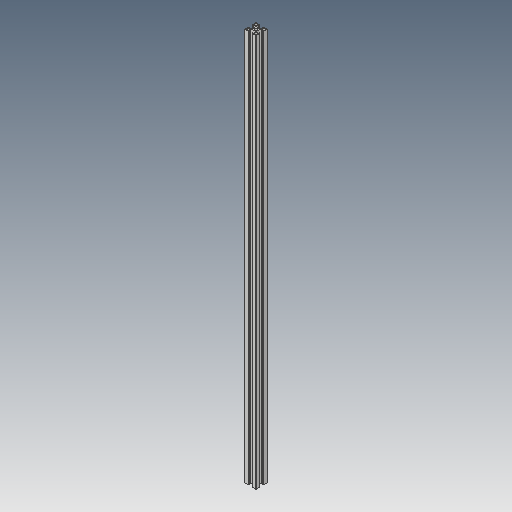
# Autodesk Inventor part: Propile_202070
Saved by Autodesk Inventor 2019 (Build 230136000, 136)
## iProperties
Created: 2019-05-03
Part Number: Propile_202070
Material: 일반
Document SubType Name: Modeling
Designer: hinmo
Density: 1 g/cm^3
Appearance: 기본값
Author: hinmo
Autodesk Inventor part; units mm, degrees
ref_plane "YZ Plane" through (0, 0, 0) normal (1, 0, 0) x (0, 1, 0)
ref_plane "XZ Plane" through (0, 0, 0) normal (0, 1, 0) x (-1, 0, 0)
ref_plane "XY Plane" through (0, 0, 0) normal (0, 0, 1) x (1, 0, 0)
sketch "스케치1" plane through (0, 0, 0) normal (0, 1, 0) x (-1, 0, 0)
  line L0 (10, 10) -> (-10, 10)
  line L1 (-10, 10) -> (-10, -10)
  line L2 (-10, -10) -> (10, -10)
  line L3 (10, -10) -> (10, 10)
  line L4 (10, 10) -> (-10, -10) construction
  line L5 (-10, 10) -> (10, -10) construction
  circle A0 centre (0, 0) radius 2.15
  line L6 (-10, 0) -> (-10, 2.65)
  line L7 (-10, 2.65) -> (-8.5, 2.65)
  line L8 (-8.5, 2.65) -> (-8.5, 4.15)
  line L9 (-8.5, 4.15) -> (-5, 4.15)
  line L10 (7, 7) -> (-7, -7) construction
  line L11 (-7, 7) -> (7, -7) construction
  circle A1 centre (-7, -7) radius 2
  circle A2 centre (-7, 7) radius 2
  circle A3 centre (7, 7) radius 2
  circle A4 centre (7, -7) radius 2
  line L12 (0, -10) -> (0, 0)
  line L13 (-10, 0) -> (-10, -2.65)
  line L14 (-10, -2.65) -> (-8.5, -2.65)
  line L15 (-8.5, -2.65) -> (-8.5, -4.15)
  line L16 (-8.5, -4.15) -> (-5, -4.15)
  arc A5 (-5, -4.15) -> (-5, 4.15) centre (-10.26, 0) ccw
  line L17 (0, 10) -> (2.65, 10)
  line L18 (2.65, 10) -> (2.65, 8.5)
  line L19 (2.65, 8.5) -> (4.15, 8.5)
  line L20 (4.15, 8.5) -> (4.15, 5)
  line L21 (0, 10) -> (-2.65, 10)
  line L22 (-2.65, 10) -> (-2.65, 8.5)
  line L23 (-2.65, 8.5) -> (-4.15, 8.5)
  line L24 (-4.15, 8.5) -> (-4.15, 5)
  arc A6 (-4.15, 5) -> (4.15, 5) centre (0, 10.26) ccw
  line L25 (8.5, -2.65) -> (8.5, -4.15)
  line L26 (10, 0) -> (10, -2.65)
  line L27 (8.5, -4.15) -> (5, -4.15)
  arc A7 (5, 4.15) -> (5, -4.15) centre (10.26, 0) ccw
  line L28 (10, -2.65) -> (8.5, -2.65)
  line L29 (8.5, 4.15) -> (5, 4.15)
  line L30 (8.5, 2.65) -> (8.5, 4.15)
  line L31 (10, 0) -> (10, 2.65)
  line L32 (10, 2.65) -> (8.5, 2.65)
  line L33 (-4.15, -8.5) -> (-4.15, -5)
  line L34 (4.15, -8.5) -> (4.15, -5)
  line L35 (2.65, -8.5) -> (4.15, -8.5)
  line L36 (-2.65, -8.5) -> (-4.15, -8.5)
  line L37 (0, -10) -> (2.65, -10)
  line L38 (2.65, -10) -> (2.65, -8.5)
  line L39 (0, -10) -> (-2.65, -10)
  line L40 (-2.65, -10) -> (-2.65, -8.5)
  arc A8 (4.15, -5) -> (-4.15, -5) centre (0, -10.26) ccw
  dimension "d6" = 20
  dimension "d7" = 20
  dimension "d8" = 4.3
  dimension "d9" = 2.65
  dimension "d10" = 1.5
  dimension "d11" = 1.5
  dimension "d12" = 3.5
  dimension "d13" = 14
  dimension "d14" = 14
  dimension "d15" = 4
  dimension "d16" = 4
  dimension "d17" = 4
  dimension "d18" = 4
  dimension "d22" = 2.65
  dimension "d23" = 1.5
  dimension "d24" = 3.5
  dimension "d25" = 6.7
  dimension "d26" = 1.5
  dimension "d27" = 2.65
  dimension "d28" = 1.5
  dimension "d29" = 1.5
  dimension "d30" = 3.5
  dimension "d31" = 2.65
  dimension "d32" = 1.5
  dimension "d33" = 3.5
  dimension "d34" = 6.7
  dimension "d35" = 1.5
  dimension "d36" = 2.65
  dimension "d37" = 1.5
  dimension "d38" = 1.5
  dimension "d39" = 3.5
  dimension "d40" = 2.65
  dimension "d41" = 1.5
  dimension "d42" = 3.5
  dimension "d43" = 6.7
  dimension "d44" = 1.5
  dimension "d45" = 2.65
  dimension "d46" = 1.5
  dimension "d47" = 1.5
  dimension "d48" = 3.5
  dimension "d49" = 2.65
  dimension "d50" = 1.5
  dimension "d51" = 3.5
  dimension "d52" = 6.7
  dimension "d53" = 1.5
  constraints: 82 end point, 21 perpendicular, 9 centre point, 8 point on circle, 5 coincident, 4 midpoint, 2 parallel, 1 horizontal, 1 vertical
  measures "d6" distance of L2.end L1.end
  measures "d7" distance of L1.end L0.end
  measures "d8" diameter of A0
  measures "d9" distance of L6.start L6.end
  measures "d10" distance of L6.end L7.end
  measures "d11" distance of L7.end L8.end
  measures "d12" distance of L8.end L9.end
  measures "d13" distance of L11.end L10.end
  measures "d14" distance of L10.end L11.start
  measures "d15" diameter of A1
  measures "d16" diameter of A2
  measures "d17" diameter of A3
  measures "d18" diameter of A4
  measures "d22" distance of L6.start L13.end
  measures "d23" distance of L14.end L15.end
  measures "d24" distance of L15.end L16.end
  measures "d25" radius of A5
  measures "d26" distance of L13.end L14.end
  measures "d27" distance of L17.start L17.end
  measures "d28" distance of L17.end L19.start
  measures "d29" distance of L19.start L19.end
  measures "d30" distance of L19.end L20.end
  measures "d31" distance of L17.start L21.end
  measures "d32" distance of L23.start L24.start
  measures "d33" distance of L24.start L24.end
  measures "d34" radius of A6
  measures "d35" distance of L21.end L23.start
  measures "d36" distance of L31.start L26.end
  measures "d37" distance of L26.end L25.start
  measures "d38" distance of L25.start L27.start
  measures "d39" distance of L27.start L27.end
  measures "d40" distance of L31.start L31.end
  measures "d41" distance of L30.start L29.start
  measures "d42" distance of L29.start L29.end
  measures "d43" radius of A7
  measures "d44" distance of L31.end L30.start
  measures "d45" distance of L37.start L39.end
  measures "d46" distance of L39.end L40.end
  measures "d47" distance of L40.end L33.start
  measures "d48" distance of L33.start L33.end
  measures "d49" distance of L37.start L38.start
  measures "d50" distance of L38.end L35.end
  measures "d51" distance of L35.end L34.end
  measures "d52" radius of A8
  measures "d53" distance of L38.start L38.end
extrude "돌출1" add sketch "스케치1" along normal blind 700 contours L3 L32 L30 L29 A7 L27 L25 L28 L2 L38 L35 L34 A8 L33 L36 L40 L1 L14 L15 L16 A5 L9 L8 L7 L0 L22 L23 L24 A6 L20 L19 L18
fillet "모깎기1" radius 0.3 12 edges at (10, 350, -10) (-10, 350, -10) (-10, 350, 10) (-10, 350, 2.65) (-10, 350, -2.65) (-2.65, 350, -10) (2.65, 350, -10) (10, 350, 10) (10, 350, 2.65) (10, 350, -2.65) (-2.65, 350, 10) (2.65, 350, 10)
